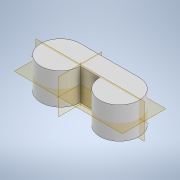
# Autodesk Inventor part: FootP
Saved by Autodesk Inventor 2021 (Build 250183000, 183)
## iProperties
Created: 2020-12-19
Part Number: FootP
Material: 一般
Document SubType Name: Modeling
Designer: Tazaki
Density: 0.865039 g/cm^3
Appearance: 既定
Mass: 500 g
Surface Area: 470 cm^2
Volume: 600 cm^3
Author: Tazaki
Autodesk Inventor part; units mm, degrees
sketch "スケッチ2" plane through (0, 0, 0) normal (0, 0, 1) x (1, 0, 0)
  line L0 (-50, 40) -> (100, 40)
  line L1 (100, 40) -> (100, -40)
  line L2 (100, -40) -> (-50, -40)
  line L3 (-50, -40) -> (-50, 40)
  point P0 (0, 0)
  point P1 (-50, 0)
  dimension "d2" = 150
  dimension "d3" = 80
  dimension "d4" = 50
  constraints: 8 end point, 2 parallel, 1 horizontal, 1 horizontal alignment, 1 midpoint, 1 perpendicular
  measures "d2" distance of L0.start L0.end
  measures "d3" distance of L2.end L0.start
  measures "d4" distance from line of point (0, 0) L3
extrude "押し出し1" add sketch "スケッチ2" against normal blind 50
sketch "スケッチ6" plane through (0, 0, 0) normal (0, 1, 0) x (-1, 0, 0)
  circle A0 centre (0, 0) radius 25
  dimension "d16" = 50
  constraints: 1 centre point, 1 coincident
  measures "d16" diameter of A0
extrude "押し出し5" [suppressed]
sketch "スケッチ7" plane through (-50, -40, -50) normal (0, -1, 0) x (1, 0, 0)
  circle A0 centre (50, 50) radius 20
  dimension "d19" = 40
  constraints: 1 centre point, 1 coincident
  measures "d19" diameter of A0
extrude "押し出し6" [suppressed]
sketch "スケッチ9" plane through (0, 0, 0) normal (0, 1, 0) x (-1, 0, 0)
  circle A0 centre (50, 0) radius 50
  circle A1 centre (-100, 0) radius 50
  line L0 (50, 0) -> (-100, 0) projected
  line L1 (-100, -50) -> (50, -50) projected
  point P0 (0, 0)
  dimension "d22" = 100
  dimension "d23" = 100
  constraints: 2 horizontal, 2 vertical alignment, 4 other
extrude "押し出し7" add sketch "スケッチ9" along normal mid plane 80 contours A0 | A1
